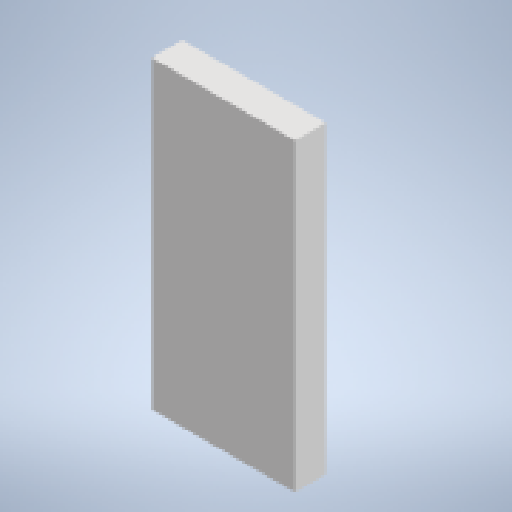
# Autodesk Inventor part: LightPipe
Saved by Autodesk Inventor 2024 (Build 280153000, 153)
## iProperties
Created: 2023-10-25
Part Number: LightPipe
Material: Generic
Document SubType Name: Modeling
Designer: jevan
Density: 1 g/cm^3
Appearance: Default
Author: jevan
Autodesk Inventor part; units mm, degrees
ref_plane "YZ Plane" through (0, 0, 0) normal (1, 0, 0) x (0, 1, 0)
ref_plane "XZ Plane" through (0, 0, 0) normal (0, 1, 0) x (-1, 0, 0)
ref_plane "XY Plane" through (0, 0, 0) normal (0, 0, 1) x (1, 0, 0)
sketch "Sketch1" plane through (0, 0, 0) normal (0, 0, 1) x (1, 0, 0)
  line L0 (0, 0) -> (3.325, 0)
  line L1 (3.325, 0) -> (3.325, 7.7)
  line L2 (3.325, 7.7) -> (0, 7.7)
  line L3 (0, 7.7) -> (0, 0)
  circle A0 centre (2.225, 6) radius 0.8
  circle A1 centre (2.225, 1.7) radius 0.8
  line L4 (3.025, 6) -> (3.025, 1.7)
  line L5 (1.425, 6) -> (1.425, 1.7)
  line L6 (2.225, 6) -> (2.225, 7.7)
  dimension "d0" = 7.7
  dimension "d2" = 1.6
  dimension "d3" = 1.6
  dimension "d4" = 1.7
  dimension "d5" = 1.7
  dimension "d10" = 1.425
  dimension "d11" = 0.3
  constraints: 14 end point, 4 point on circle, 3 tangent, 3 vertical, 2 centre point, 2 parallel, 2 perpendicular, 1 horizontal, 1 point on line
  measures "d0" distance of L0.end L1.end
  measures "d2" diameter of A0
  measures "d3" diameter of A1
  measures "d4" distance from line of L2 L6.start
  measures "d5" distance from line of L0 A1.centre
  measures "d10" distance between parallel lines of L3 L5
  measures "d11" distance between parallel lines of L4 L1
extrude "Extrusion1" add sketch "Sketch1" along normal blind 0.8 contours A0 | L3 L2 L1 L0 | L4 A1 L5 A0 | A1
extrude "Extrusion2" add sketch "Sketch1" against normal blind 0.9 contours A0 | L4 A1 L5 A0 | A1
body "Solid1"
